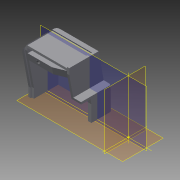
# Autodesk Inventor part: KarosserieDachTeil3
Saved by Autodesk Inventor 2015 (Build 190159000, 159)
## iProperties
Created: 2018-12-14
Part Number: KarosserieDachTeil3
Material: Generisch
Document SubType Name: Modeling
Designer: Boris
Density: 1 g/cm^3
Appearance: Vorgabe
Author: Boris
Autodesk Inventor part; units mm, degrees
sketch "Skizze2" plane through (0, 0, 0) normal (0, 0, 1) x (1, 0, 0)
  line L0 (-77, 13.5) -> (-28, 13.5)
  line L1 (-28, 13.5) -> (-28, -5.5)
  line L2 (-77, -13.5) -> (-77, 13.5)
  line L3 (-92.4, 0) -> (15.4, 0) projected
  line L4 (0, 18.9) -> (0, -18.9) projected
  line L5 (-73, 9.5) -> (-73, -13.5)
  line L6 (-73, 9.5) -> (-31, 9.5)
  line L7 (-31, 9.5) -> (-31, -5.5)
  line L8 (-31, -5.5) -> (-28, -5.5)
  line L9 (-73, -13.5) -> (-77, -13.5)
  point P0 (0, 0)
  dimension "d4" = 28
  dimension "d5" = 4
  dimension "d6" = 4
  dimension "d7" = 3
  dimension "d8" = 19
  dimension "d9" = 49
  dimension "d10" = 13.5
  dimension "d11" = 13.5
  constraints: 16 end point, 4 perpendicular, 2 horizontal, 2 parallel
  measures "d4" distance between parallel lines of L4 L1
  measures "d5" distance between parallel lines of L2 L5
  measures "d6" distance between parallel lines of L6 L0
  measures "d7" distance between parallel lines of L1 L7
  measures "d8" distance between parallel lines of L8 L0
  measures "d9" distance of L0.start L0.end
  measures "d10" distance between parallel lines of L3 L0
  measures "d11" distance between parallel lines of L3 L9
sketch "Skizze3" plane through (0, 0, 0) normal (1, 0, 0) x (0, 1, 0)
  line L0 (7.1869, 0) -> (7.1869, 15.874)
  line L1 (7.1869, 15.874) -> (1.0023, 49.9056)
  line L2 (7.1869, 15.874) -> (41.7759, 15.874) construction
  line L3 (-8.3552, 0) -> (50.1311, 0) projected
  point P0 (0, 0)
  dimension "d12" = 15.874
  dimension "d13" = 34.589
  dimension "d14" = 100.3
  dimension "d15" = 0
  constraints: 6 end point, 1 equal length, 1 horizontal, 1 vertical
  measures "d12" distance of L0.start L0.end
  measures "d13" distance of L0.end L1.end
  measures "d14" angle of L2 L1
  measures "d15" distance from line of L3 L0.start
sweep "Sweeping1" add profiles "Skizze2" path "Skizze3" path curves L0 L1 contours L0 L1 L3 L7 L6 L5 L2 | L3 L5 L9 L2 | L1 L8 L7 L3
sketch "Skizze4" plane through (-77, 13.5, 0) normal (0, 1, 0) x (1, 0, 0)
  circle A0 centre (16.5, -10.409) radius 1.5
  line L0 (0, 0) -> (0, -16.443) projected
  line L1 (0, 0) -> (49, 0) projected
  point P0 (77, 0)
  dimension "d18" = 3
  dimension "d19" = 16.5
  dimension "d20" = 10.409
  constraints: 1 centre point
  measures "d18" diameter of A0
  measures "d19" distance from line of L0 A0.centre
  measures "d20" distance from line of L1 A0.centre
extrude "Extrusion1" cut sketch "Skizze4" against normal blind 5
sketch "Skizze6" plane through (-77, -13.5, 0) normal (-1, 0, 0) x (0, 0, 1)
  line L0 (46.2067, -5.8512) -> (8.2228, 0)
  line L1 (8.2228, 0) -> (14.0095, 0)
  line L2 (0, 0) -> (14.0095, 0) projected
  line L3 (14.0095, 0) -> (46.2067, -5.8512)
  point P0 (0, 13.5)
  dimension "d24" = 38.432
  constraints: 6 end point, 1 collinear
  measures "d24" distance of L0.start L0.end
extrude "Extrusion2" add sketch "Skizze6" against normal up to surface (4 mm away)
sketch "Skizze7" plane through (-77, -13.5, 0) normal (-1, 0, 0) x (0, 0, 1)
  line L0 (8.2228, 0) -> (45.982, -7.0714)
  line L1 (46.2067, -5.8512) -> (45.982, -7.0714)
  line L2 (8.2228, 0) -> (46.2067, -5.8512) projected
  point P0 (0, 13.5)
  point P1 (51.0344, 20.7137)
  dimension "d27" = 1.85
  constraints: 4 end point, 1 point on line
  measures "d27" angle of L2 L0
extrude "Extrusion3" add sketch "Skizze7" against normal blind 4
sketch "Skizze8" plane through (-77, -13.5, 0) normal (-1, 0, 0) x (0, 0, 1)
  line L0 (45.982, -7.0714) -> (45.982, 21.6319)
  line L1 (45.982, 21.6319) -> (55.7494, 19.8568)
  line L2 (16.443, 27) -> (51.0344, 20.7137) projected
  line L3 (45.982, -7.0714) -> (56.0602, 20.7137)
  point P0 (0, 13.5)
  constraints: 6 end point, 1 collinear, 1 point on line, 1 vertical
extrude "Extrusion4" cut sketch "Skizze8" against normal blind 50
sketch "Skizze9" plane through (-73, -13.5, 0) normal (1, 0, 0) x (0, 0, -1)
  line L0 (-45.982, -7.0714) -> (-8.2228, 0) projected
  line L1 (0, 0) -> (-8.2228, 0) projected
  line L2 (-45.6631, -5.9943) -> (-8.3156, 1)
  line L3 (-8.3156, 1) -> (0, 1)
  line L4 (-45.6631, -5.9943) -> (-45.4813, -6.9776)
  line L5 (0, 0) -> (0, 1)
  point P0 (0, 13.5)
  dimension "d32" = 1
  constraints: 8 end point, 1 point on line, 1 other
  measures "d32" distance between parallel lines of L0 L2
extrude "Extrusion5" cut sketch "Skizze9" against normal blind 1.906
sketch "Skizze10" plane through (-73, 9.5, 16.0825) normal (1, 0, 0) x (0, 0, -1)
  line L0 (-30.0127, -30.2379) -> (-24.3951, -30.2379)
  line L1 (-24.3951, -30.2379) -> (-24.3951, -28.0504)
  line L2 (-24.3951, -28.0504) -> (-30.0127, -28.0504)
  line L3 (-30.0127, -28.0504) -> (-30.0127, -30.2379)
  point P0 (16.0825, -9.5)
  constraints: 8 end point, 1 horizontal, 1 parallel, 1 perpendicular, 1 vertical
extrude "Extrusion6" cut sketch "Skizze10" against normal up to surface (1.906 mm away)
sketch "Skizze14" plane through (-77, 13.5, 0) normal (0, 1, 0) x (1, 0, 0)
  circle A0 centre (13, -35.7606) radius 1.5
  line L0 (0, -16.443) -> (0, -45.982) projected
  point P0 (77, 0)
  dimension "d46" = 3
  dimension "d48" = 13
  constraints: 1 centre point
  measures "d46" diameter of A0
  measures "d48" distance from line of L0 A0.centre
extrude "Extrusion10" cut sketch "Skizze14" against normal blind 8
sketch "Skizze15" plane through (0, 0, 0) normal (0, 1, 0) x (-1, 0, 0)
  line L0 (31, 38.5351) -> (31, 32.5351)
  line L1 (31, 32.5351) -> (73, 32.5351)
  line L2 (73, 32.5351) -> (73, 38.5351)
  line L3 (73, 38.5351) -> (31, 38.5351)
  circle A0 centre (64, 35.7606) radius 1.5 projected
  point P0 (0, 0)
  constraints: 8 end point, 1 parallel
extrude "Extrusion11" add sketch "Skizze15" along normal up to surface starts on plane at (-73, -19.4943, 45.6631) facing (0, 0.982912, 0.1840759) surface through (-73, 9.5, 16.0825) normal (0, -0.983885, -0.1788022)
chamfer "Fase1" distance 20 distance2 8 1 edges at (-31, -17.5976, 35.5351) measured on face at (-31.5, -17.5976, 35.5351)
thread "Gewinde1"
thread "Gewinde2"
sketch "Skizze17" plane through (-73, -18.5504, 45.982) normal (1, 0, 0) x (0, 0, -1)
  line L0 (0, 0) -> (5.3588, 0) projected
  line L1 (1.0305, 0) -> (1.0305, 22.8041)
  line L2 (7.4469, 23.9701) -> (0, 22.6168) projected
  line L3 (1.0305, 0) -> (23.8345, 0) construction
  line L4 (1.0305, 0) -> (3.0305, 0)
  line L5 (3.0305, 0) -> (3.0305, 23.1675)
  line L6 (3.0305, 23.1675) -> (1.0305, 22.8041)
  point P0 (45.982, 18.5504)
  dimension "d66" = 90
  dimension "d67" = 2
  dimension "d68" = 90
  constraints: 10 end point, 4 point on line, 1 collinear, 1 horizontal, 1 perpendicular
  measures "d66" angle of L3 L1
  measures "d67" distance of L1.start L4.end
  measures "d68" angle of L5 L4
extrude "Extrusion13" add sketch "Skizze17" along normal up to surface (42 mm away)
sketch "Skizze18" plane through (-77, -20.5714, 45.982) normal (0, 0, 1) x (1, 0, 0)
  line L0 (57, 2.021) -> (42, 2.021)
  line L1 (4, 2.021) -> (46, 2.021) projected
  line L2 (42, 2.021) -> (42, 42.021)
  line L3 (42, 42.021) -> (57, 42.021)
  line L4 (57, 42.021) -> (57, 2.021)
  line L5 (49, 28.7033) -> (49, 9.3921) projected
  point P0 (77, 20.5714)
  dimension "d71" = 15
  dimension "d72" = 40
  dimension "d73" = 7
  constraints: 8 end point, 3 perpendicular, 1 point on line
  measures "d71" distance of L0.start L0.end
  measures "d72" distance of L0.end L2.end
  measures "d73" distance between parallel lines of L2 L5
extrude "Extrusion14" cut sketch "Skizze18" against normal blind 25
sketch "Skizze19" plane through (-77, 13.5, 0) normal (0, 1, 0) x (1, 0, 0)
  line L0 (42, -20.982) -> (49, -20.982) projected
  line L1 (42, -45.982) -> (42, -20.982) projected
  line L2 (40, -45.982) -> (40, -18.982)
  line L3 (40, -18.982) -> (49, -18.982)
  line L4 (42, -45.982) -> (40, -45.982)
  line L5 (42, -45.982) -> (4, -45.982) projected
  line L6 (49, -18.982) -> (49, -20.982)
  line L7 (49, -14.7306) -> (49, -20.982) projected
  point P0 (77, 0)
  dimension "d76" = 2
  constraints: 8 end point, 2 collinear, 1 other
  measures "d76" distance between parallel lines of L1 L2
extrude "Extrusion15" add sketch "Skizze19" against normal up to surface (32.0504 mm away)
sketch "Skizze20" plane through (-35, -18.5504, 45.982) normal (1, 0, 0) x (0, 0, -1)
  line L0 (0, 26.6823) -> (27, 31.589) projected
  line L1 (27, 32.0504) -> (27, 31.589) projected
  line L2 (25, 32.0504) -> (27, 32.0504) projected
  line L3 (0, 32.0504) -> (25, 32.0504) projected
  line L4 (0, 0) -> (0, 32.0504) projected
  point P0 (45.982, 18.5504)
extrude "Extrusion16" cut sketch "Skizze20" along normal mid plane 23
sketch "Skizze21" plane through (-35, -18.5504, 45.982) normal (1, 0, 0) x (0, 0, -1)
  line L0 (7.4469, 0.3911) -> (13.4469, 1.5147) projected
  line L1 (13.4469, 1.5147) -> (37.6664, 6.0504) projected
  line L2 (37.6664, 6.0504) -> (37.6664, -7.7967)
  line L3 (37.6664, -7.7967) -> (-7.4675, -7.7967)
  line L4 (-7.4675, -7.7967) -> (-7.4675, -2.402)
  line L5 (37.6664, 6.0504) -> (-7.4675, -2.402)
  point P0 (45.982, 18.5504)
  constraints: 8 end point, 2 perpendicular, 1 point on line, 1 vertical
extrude "Extrusion17" cut sketch "Skizze21" along normal mid plane 23
chamfer "Fase2" distance 7 distance2 4 1 edges at (-77, -6.2198, 45.982) measured on face at (-77, -6.2198, 45.482)
sketch "Skizze22" plane through (-77, 13.5, 0) normal (0, 1, 0) x (1, 0, 0)
  circle A0 centre (13, -35.7606) radius 1.5 projected
  circle A1 centre (13, -35.7606) radius 2.5
  point P0 (77, 0)
  dimension "d86" = 1
  constraints: 1 centre point
  measures "d86" radial gap between concentric circles of A0 A1
extrude "Extrusion18" cut sketch "Skizze22" against normal blind 4
sketch "Skizze23" plane through (-64, 9.5, 35.7606) normal (0, 1, 0) x (1, 0, 0)
  circle A0 centre (0, 0) radius 2.5 projected
  circle A1 centre (0, 0) radius 1.5 projected
  point P0 (64, 35.7606)
extrude "Extrusion19" add sketch "Skizze23" along normal blind 1
fillet "Rundung5" radius 3 3 edges at (-77, 13.5, 8.2215) (-77, 11.452, 27.7125) (-75, 8.7679, 42.482)
fillet "Rundung6" radius 3 3 edges at (-76.997, 6.4893, 38.9872) (-76.025, 8.5826, 39.1027) (-77, -6.4528, 38.982)
fillet "Rundung7" radius 2 2 edges at (-28, 13.5, 8.2215) (-28, 13.0876, 18.7125)
